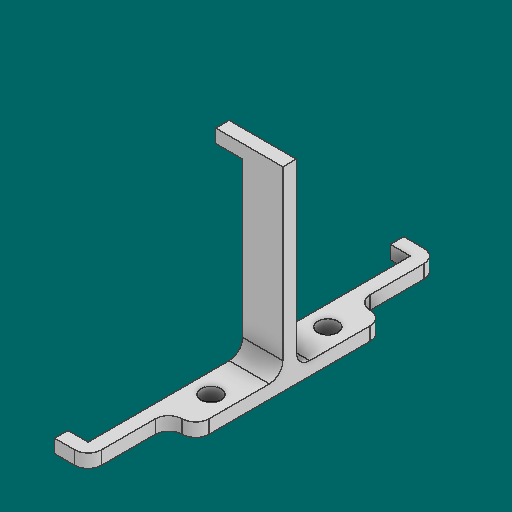
# Autodesk Inventor part: battery_holder_1
Saved by Autodesk Inventor 2026.1 (Build 301233000, 233)
## iProperties
Created: 2025-12-03
Part Number: battery_holder_1
Material: Generic
Document SubType Name: Modeling
Designer: emanuel
Density: 1 g/cm^3
Appearance: Default
Author: emanuel
Autodesk Inventor part; units mm, degrees
ref_plane "YZ Plane" through (0, 0, 0) normal (1, 0, 0) x (0, 1, 0)
ref_plane "XZ Plane" through (0, 0, 0) normal (0, 1, 0) x (-1, 0, 0)
ref_plane "XY Plane" through (0, 0, 0) normal (0, 0, 1) x (1, 0, 0)
sketch "Sketch1" plane through (0, 0, 0) normal (0, 1, 0) x (-1, 0, 0)
  line L0 (0, 0) -> (6, 0)
  line L1 (6, 0) -> (6, -52)
  line L2 (6, -52) -> (0, -52)
  line L3 (0, -52) -> (0, 0)
  line L4 (6, 0) -> (9, 0)
  line L5 (9, 0) -> (9, -2)
  line L6 (9, -2) -> (6, -2)
  line L7 (6, -2) -> (6, 0)
  line L8 (6, -52) -> (9, -52)
  line L9 (9, -52) -> (9, -50)
  line L10 (9, -50) -> (6, -50)
  line L11 (6, -50) -> (6, -52)
  line L12 (0, 0) -> (4, 0)
  line L13 (4, 0) -> (4, -12)
  line L14 (4, -12) -> (0, -12)
  line L15 (0, -12) -> (0, 0)
  line L16 (0, -52) -> (4, -52)
  line L17 (4, -52) -> (4, -40)
  line L18 (4, -40) -> (0, -40)
  line L19 (0, -40) -> (0, -52)
  line L20 (0, -26) -> (3, -26)
  line L21 (3, -26) -> (3, -34.7)
  line L22 (3, -34.7) -> (3, -17.3)
  circle A0 centre (3, -17.3) radius 1.5
  circle A1 centre (3, -34.7) radius 1.5
  point P0 (0, -40)
  point P1 (6, -50)
  point P2 (6, -2)
  dimension "d0" = 6
  dimension "d1" = 52
  dimension "d2" = 3
  dimension "d3" = 2
  dimension "d4" = 3
  dimension "d5" = 2
  dimension "d6" = 4
  dimension "d7" = 12
  dimension "d8" = 4
  dimension "d9" = 12
  dimension "d10" = 3
  dimension "d11" = 8.7
  dimension "d12" = 17.4
  dimension "d13" = 3
  dimension "d14" = 3
  constraints: 46 end point, 10 parallel, 6 horizontal, 6 perpendicular, 2 centre point, 2 coincident, 1 midpoint, 1 point on line
  measures "d0" distance of L1.end L2.end
  measures "d1" distance of L0.end L1.end
  measures "d2" distance of L5.end L6.end
  measures "d3" distance of L4.end L5.end
  measures "d4" distance of L10.end L9.end
  measures "d5" distance of L9.end L8.end
  measures "d6" distance of L13.end L14.end
  measures "d7" distance of L12.end L13.end
  measures "d8" distance of L18.end L17.end
  measures "d9" distance of L17.end L16.end
  measures "d10" distance of L20.start L20.end
  measures "d11" distance of L20.end L21.end
  measures "d12" distance of L21.end L22.end
  measures "d13" diameter of A0
  measures "d14" diameter of A1
extrude "Extrusion1" add sketch "Sketch1" along normal blind 2 contours L0 L1 L2 L17 L18 L3 L14 L13 | L4 L5 L6 L1 | L10 L9 L8 L1
sketch "Sketch2" plane through (0, 2, 0) normal (0, 1, 0) x (1, 0, 0)
  line L0 (0, 12) -> (0, 40) projected
  line L1 (0, 26) -> (-6, 26)
  line L2 (-6, 50) -> (-6, 2) projected
  line L3 (0, 25) -> (-6, 25)
  line L4 (-6, 25) -> (-6, 27)
  line L5 (-6, 27) -> (0, 27)
  line L6 (0, 27) -> (0, 25)
  line L7 (0, 25) -> (-6, 27) construction
  line L8 (-6, 25) -> (0, 27) construction
  point P0 (0, 0)
  point P1 (-3, 26)
  point P2 (0, 25)
  point P3 (0, 27)
  dimension "d17" = 2
  constraints: 14 end point, 5 midpoint, 2 parallel, 1 horizontal, 1 perpendicular, 1 point on line
  measures "d17" distance of L3.end L4.end
extrude "Extrusion2" add sketch "Sketch2" along normal blind 27
sketch "Sketch3" plane through (-6, 0, -50) normal (-1, 0, 0) x (0, 0, 1)
  line L0 (23, 29) -> (25, 29) projected
  line L1 (25, 2) -> (25, 29) projected
  line L2 (23, 29) -> (25, 29)
  line L3 (25, 29) -> (25, 27)
  line L4 (25, 27) -> (23, 27)
  line L5 (23, 27) -> (23, 29)
  point P0 (50, 0)
  dimension "d20" = 2
  constraints: 8 end point, 2 parallel, 1 horizontal, 1 perpendicular, 1 point on line
  measures "d20" distance of L2.end L3.end
extrude "Extrusion3" add sketch "Sketch3" along normal blind 4
fillet "Fillet1" radius 2 8 edges at (-3, 2, -25) (-3, 2, -27) (-4, 1, -12) (-4, 1, 0) (-4, 1, -52) (0, 1, -40) (0, 1, -12) (-4, 1, -40)
body "Solid1"
